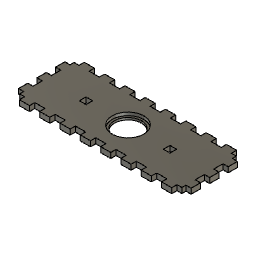
Top_of_Box-v3 (Autodesk Fusion 360 design; units mm, degrees)
Autodesk Fusion 360 part; units mm, degrees
sketch "Sketch1" plane through (0, 0, 0) normal (0, 0, 1) x (1, 0, 0)
  line L0 (0, 0) -> (165, 0)
  line L1 (165, 0) -> (165, 62)
  line L2 (165, 62) -> (0, 62)
  line L3 (0, 62) -> (0, 0)
  line L4 (0, 62) -> (9.7059, 62)
  line L5 (9.7059, 62) -> (9.7059, 57)
  line L6 (9.7059, 57) -> (0, 57)
  line L7 (0, 57) -> (0, 62)
  line L8 (9.7059, 62) -> (19.4118, 62)
  line L9 (19.4118, 62) -> (19.4118, 57)
  line L10 (19.4118, 57) -> (9.7059, 57)
  line L11 (9.7059, 57) -> (9.7059, 62)
  line L12 (19.4118, 62) -> (29.1176, 62)
  line L13 (29.1176, 62) -> (29.1176, 57)
  line L14 (29.1176, 57) -> (19.4118, 57)
  line L15 (19.4118, 57) -> (19.4118, 62)
  line L16 (29.1176, 62) -> (38.8235, 62)
  line L17 (38.8235, 62) -> (38.8235, 57)
  line L18 (38.8235, 57) -> (29.1176, 57)
  line L19 (29.1176, 57) -> (29.1176, 62)
  line L20 (38.8235, 62) -> (48.5294, 62)
  line L21 (48.5294, 62) -> (48.5294, 57)
  line L22 (48.5294, 57) -> (38.8235, 57)
  line L23 (38.8235, 57) -> (38.8235, 62)
  line L24 (48.5294, 62) -> (58.2353, 62)
  line L25 (58.2353, 62) -> (58.2353, 57)
  line L26 (58.2353, 57) -> (48.5294, 57)
  line L27 (48.5294, 57) -> (48.5294, 62)
  line L28 (58.2353, 62) -> (67.9412, 62)
  line L29 (67.9412, 62) -> (67.9412, 57)
  line L30 (67.9412, 57) -> (58.2353, 57)
  line L31 (58.2353, 57) -> (58.2353, 62)
  line L32 (67.9412, 62) -> (77.6471, 62)
  line L33 (77.6471, 62) -> (77.6471, 57)
  line L34 (77.6471, 57) -> (67.9412, 57)
  line L35 (67.9412, 57) -> (67.9412, 62)
  line L36 (77.6471, 62) -> (87.3529, 62)
  line L37 (87.3529, 62) -> (87.3529, 57)
  line L38 (87.3529, 57) -> (77.6471, 57)
  line L39 (77.6471, 57) -> (77.6471, 62)
  line L40 (87.3529, 62) -> (97.0588, 62)
  line L41 (97.0588, 62) -> (97.0588, 57)
  line L42 (97.0588, 57) -> (87.3529, 57)
  line L43 (87.3529, 57) -> (87.3529, 62)
  line L44 (97.0588, 62) -> (106.7647, 62)
  line L45 (106.7647, 62) -> (106.7647, 57)
  line L46 (106.7647, 57) -> (97.0588, 57)
  line L47 (97.0588, 57) -> (97.0588, 62)
  line L48 (106.7647, 62) -> (116.4706, 62)
  line L49 (116.4706, 62) -> (116.4706, 57)
  line L50 (116.4706, 57) -> (106.7647, 57)
  line L51 (106.7647, 57) -> (106.7647, 62)
  line L52 (116.4706, 62) -> (126.1765, 62)
  line L53 (126.1765, 62) -> (126.1765, 57)
  line L54 (126.1765, 57) -> (116.4706, 57)
  line L55 (116.4706, 57) -> (116.4706, 62)
  line L56 (126.1765, 62) -> (135.8824, 62)
  line L57 (135.8824, 62) -> (135.8824, 57)
  line L58 (135.8824, 57) -> (126.1765, 57)
  line L59 (126.1765, 57) -> (126.1765, 62)
  line L60 (135.8824, 62) -> (145.5882, 62)
  line L61 (145.5882, 62) -> (145.5882, 57)
  line L62 (145.5882, 57) -> (135.8824, 57)
  line L63 (135.8824, 57) -> (135.8824, 62)
  line L64 (145.5882, 62) -> (155.2941, 62)
  line L65 (155.2941, 62) -> (155.2941, 57)
  line L66 (155.2941, 57) -> (145.5882, 57)
  line L67 (145.5882, 57) -> (145.5882, 62)
  line L68 (155.2941, 62) -> (165, 62)
  line L69 (165, 62) -> (165, 57)
  line L70 (165, 57) -> (155.2941, 57)
  line L71 (155.2941, 57) -> (155.2941, 62)
  line L72 (0, 62) -> (5, 62)
  line L73 (5, 62) -> (5, 53.1429)
  line L74 (5, 53.1429) -> (0, 53.1429)
  line L75 (0, 53.1429) -> (0, 62)
  line L76 (5, 44.2857) -> (0, 44.2857)
  line L77 (5, 53.1429) -> (5, 44.2857)
  line L78 (0, 44.2857) -> (0, 53.1429)
  line L79 (0, 53.1429) -> (5, 53.1429)
  line L80 (5, 35.4286) -> (0, 35.4286)
  line L81 (5, 44.2857) -> (5, 35.4286)
  line L82 (0, 35.4286) -> (0, 44.2857)
  line L83 (0, 44.2857) -> (5, 44.2857)
  line L84 (5, 26.5714) -> (0, 26.5714)
  line L85 (5, 35.4286) -> (5, 26.5714)
  line L86 (0, 26.5714) -> (0, 35.4286)
  line L87 (0, 35.4286) -> (5, 35.4286)
  line L88 (5, 17.7143) -> (0, 17.7143)
  line L89 (5, 26.5714) -> (5, 17.7143)
  line L90 (0, 17.7143) -> (0, 26.5714)
  line L91 (0, 26.5714) -> (5, 26.5714)
  line L92 (5, 8.8571) -> (0, 8.8571)
  line L93 (5, 17.7143) -> (5, 8.8571)
  line L94 (0, 8.8571) -> (0, 17.7143)
  line L95 (0, 17.7143) -> (5, 17.7143)
  line L96 (5, 0) -> (0, 0)
  line L97 (5, 8.8571) -> (5, 0)
  line L98 (0, 0) -> (0, 8.8571)
  line L99 (0, 8.8571) -> (5, 8.8571)
  line L100 (0, 0) -> (9.7059, 0)
  line L101 (9.7059, 0) -> (9.7059, 5)
  line L102 (9.7059, 5) -> (0, 5)
  line L103 (0, 5) -> (0, 0)
  line L104 (9.7059, 0) -> (19.4118, 0)
  line L105 (19.4118, 0) -> (19.4118, 5)
  line L106 (9.7059, 5) -> (9.7059, 0)
  line L107 (19.4118, 5) -> (9.7059, 5)
  line L108 (19.4118, 0) -> (29.1176, 0)
  line L109 (29.1176, 0) -> (29.1176, 5)
  line L110 (19.4118, 5) -> (19.4118, 0)
  line L111 (29.1176, 5) -> (19.4118, 5)
  line L112 (29.1176, 0) -> (38.8235, 0)
  line L113 (38.8235, 0) -> (38.8235, 5)
  line L114 (29.1176, 5) -> (29.1176, 0)
  line L115 (38.8235, 5) -> (29.1176, 5)
  line L116 (38.8235, 0) -> (48.5294, 0)
  line L117 (48.5294, 0) -> (48.5294, 5)
  line L118 (38.8235, 5) -> (38.8235, 0)
  line L119 (48.5294, 5) -> (38.8235, 5)
  line L120 (48.5294, 0) -> (58.2353, 0)
  line L121 (58.2353, 0) -> (58.2353, 5)
  line L122 (48.5294, 5) -> (48.5294, 0)
  line L123 (58.2353, 5) -> (48.5294, 5)
  line L124 (58.2353, 0) -> (67.9412, 0)
  line L125 (67.9412, 0) -> (67.9412, 5)
  line L126 (58.2353, 5) -> (58.2353, 0)
  line L127 (67.9412, 5) -> (58.2353, 5)
  line L128 (67.9412, 0) -> (77.6471, 0)
  line L129 (77.6471, 0) -> (77.6471, 5)
  line L130 (67.9412, 5) -> (67.9412, 0)
  line L131 (77.6471, 5) -> (67.9412, 5)
  line L132 (77.6471, 0) -> (87.3529, 0)
  line L133 (87.3529, 0) -> (87.3529, 5)
  line L134 (77.6471, 5) -> (77.6471, 0)
  line L135 (87.3529, 5) -> (77.6471, 5)
  line L136 (87.3529, 0) -> (97.0588, 0)
  line L137 (97.0588, 0) -> (97.0588, 5)
  line L138 (87.3529, 5) -> (87.3529, 0)
  line L139 (97.0588, 5) -> (87.3529, 5)
  line L140 (97.0588, 0) -> (106.7647, 0)
  line L141 (106.7647, 0) -> (106.7647, 5)
  line L142 (97.0588, 5) -> (97.0588, 0)
  line L143 (106.7647, 5) -> (97.0588, 5)
  line L144 (106.7647, 0) -> (116.4706, 0)
  line L145 (116.4706, 0) -> (116.4706, 5)
  line L146 (106.7647, 5) -> (106.7647, 0)
  line L147 (116.4706, 5) -> (106.7647, 5)
  line L148 (116.4706, 0) -> (126.1765, 0)
  line L149 (126.1765, 0) -> (126.1765, 5)
  line L150 (116.4706, 5) -> (116.4706, 0)
  line L151 (126.1765, 5) -> (116.4706, 5)
  line L152 (126.1765, 0) -> (135.8824, 0)
  line L153 (135.8824, 0) -> (135.8824, 5)
  line L154 (126.1765, 5) -> (126.1765, 0)
  line L155 (135.8824, 5) -> (126.1765, 5)
  line L156 (135.8824, 0) -> (145.5882, 0)
  line L157 (145.5882, 0) -> (145.5882, 5)
  line L158 (135.8824, 5) -> (135.8824, 0)
  line L159 (145.5882, 5) -> (135.8824, 5)
  line L160 (145.5882, 0) -> (155.2941, 0)
  line L161 (155.2941, 0) -> (155.2941, 5)
  line L162 (145.5882, 5) -> (145.5882, 0)
  line L163 (155.2941, 5) -> (145.5882, 5)
  line L164 (155.2941, 0) -> (165, 0)
  line L165 (165, 0) -> (165, 5)
  line L166 (155.2941, 5) -> (155.2941, 0)
  line L167 (165, 5) -> (155.2941, 5)
  line L168 (165, 62) -> (160, 62)
  line L169 (160, 62) -> (160, 53.1429)
  line L170 (160, 53.1429) -> (165, 53.1429)
  line L171 (165, 53.1429) -> (165, 62)
  line L172 (160, 53.1429) -> (160, 44.2857)
  line L173 (160, 44.2857) -> (165, 44.2857)
  line L174 (160, 44.2857) -> (160, 35.4286)
  line L175 (160, 35.4286) -> (165, 35.4286)
  line L176 (160, 35.4286) -> (160, 26.5714)
  line L177 (160, 26.5714) -> (165, 26.5714)
  line L178 (160, 26.5714) -> (160, 17.7143)
  line L179 (160, 17.7143) -> (165, 17.7143)
  line L180 (160, 17.7143) -> (160, 8.8571)
  line L181 (160, 8.8571) -> (165, 8.8571)
  line L182 (160, 8.8571) -> (160, 0)
  line L183 (160, 0) -> (165, 0)
  dimension "d4" = 165
  dimension "d5" = 62
  dimension "d6" = 9.7059
  dimension "d7" = 5
  dimension "d10" = 155.2941
  dimension "d11" = 0
  dimension "d12" = 5
  dimension "d13" = 8.8571
  dimension "d16" = 0
  dimension "d17" = -53.1429
  dimension "d18" = 9.7059
  dimension "d19" = 5
  dimension "d22" = 155.2941
  dimension "d23" = 0
  dimension "d24" = 5
  dimension "d25" = 8.8571
  dimension "d28" = 0
  dimension "d29" = -53.1429
  constraint horizontal L0
  constraint vertical L1
  constraint horizontal L2
  constraint vertical L3
  constraint coincident L0.start L3.end
  constraint horizontal L4
  constraint vertical L5
  constraint horizontal L6
  constraint vertical L7
  constraint horizontal L72
  constraint vertical L73
  constraint horizontal L74
  constraint vertical L75
  measures "d4" distance of L0.start L0.end
  measures "d5" distance of L0.start L2.end
  measures "d6" distance of L2.end L4.end
  measures "d7" distance of L2.end L6.end
  measures "d12" distance of L2.end L72.end
  measures "d13" distance of L2.end L74.end
  measures "d18" distance of L0.start L100.end
  measures "d19" distance of L0.start L102.end
  measures "d24" distance of L1.end L168.end
  measures "d25" distance of L1.end L170.end
extrude "Extrude1" add sketch "Sketch1" along normal blind 5 contours L0 L101 L104 L105 L106 L107 L110 | L6 L10 L14 L18 L22 L26 L30 L34 L38 L42 L46 L50 L54 L58 L62 L66 L70 L73 L77 L81 L85 L89 L93 L97 L102 L107 L111 L115 L119 L123 L127 L131 L135 L139 L143 L147 L151 L155 L159 L163 L167 L169 L172 L174 L176 L178 L180 L182 | L3 L88 L92 L93 L94 L95 L99 | L0 L109 L112 L113 L114 L115 L118 | L3 L80 L84 L85 L86 L87 L91 | L0 L117 L120 L121 L122 L123 L126 | L3 L74 L76 L77 L78 L79 L83 | L0 L125 L128 L129 L130 L131 L134 | L0 L133 L136 L137 L138 L139 L142 | L2 L5 L8 L9 L10 L11 L15 | L0 L141 L144 L145 L146 L147 L150 | L2 L13 L16 L17 L18 L19 L23 | L0 L149 L152 L153 L154 L155 L158 | L2 L21 L24 L25 L26 L27 L31 | L0 L157 L160 L161 L162 L163 L166 | L2 L29 L32 L33 L34 L35 L39 | L2 L37 L40 L41 L42 L43 L47 | L1 L179 L180 L181 | L2 L45 L48 L49 L50 L51 L55 | L1 L175 L176 L177 | L2 L53 L56 L57 L58 L59 L63 | L1 L170 L172 L173 | L2 L61 L64 L65 L66 L67 L71
sketch "Sketch2" plane through (0, 0, 5) normal (0, 0, 1) x (-1, 0, 0)
  line L0 (-165, -8.8571) -> (-165, -17.7143)
  line L1 (-165, -17.7143) -> (-160, -17.7143)
  line L2 (-160, -17.7143) -> (-160, -26.5714)
  line L3 (-160, -26.5714) -> (-165, -26.5714)
  line L4 (-165, -26.5714) -> (-165, -35.4286)
  line L5 (-165, -35.4286) -> (-160, -35.4286)
  line L6 (-160, -35.4286) -> (-160, -44.2857)
  line L7 (-160, -44.2857) -> (-165, -44.2857)
  line L8 (-165, -44.2857) -> (-165, -53.1429)
  line L9 (-165, -53.1429) -> (-160, -53.1429)
  line L10 (-160, -53.1429) -> (-160, -57)
  line L11 (-160, -57) -> (-155.2941, -57)
  line L12 (-155.2941, -57) -> (-155.2941, -62)
  line L13 (-155.2941, -62) -> (-145.5882, -62)
  line L14 (-145.5882, -62) -> (-145.5882, -57)
  line L15 (-145.5882, -57) -> (-135.8824, -57)
  line L16 (-135.8824, -57) -> (-135.8824, -62)
  line L17 (-135.8824, -62) -> (-126.1765, -62)
  line L18 (-126.1765, -62) -> (-126.1765, -57)
  line L19 (-126.1765, -57) -> (-116.4706, -57)
  line L20 (-116.4706, -57) -> (-116.4706, -62)
  line L21 (-116.4706, -62) -> (-106.7647, -62)
  line L22 (-106.7647, -62) -> (-106.7647, -57)
  line L23 (-106.7647, -57) -> (-97.0588, -57)
  line L24 (-97.0588, -57) -> (-97.0588, -62)
  line L25 (-97.0588, -62) -> (-87.3529, -62)
  line L26 (-87.3529, -62) -> (-87.3529, -57)
  line L27 (-87.3529, -57) -> (-77.6471, -57)
  line L28 (-77.6471, -57) -> (-77.6471, -62)
  line L29 (-77.6471, -62) -> (-67.9412, -62)
  line L30 (-67.9412, -62) -> (-67.9412, -57)
  line L31 (-67.9412, -57) -> (-58.2353, -57)
  line L32 (-58.2353, -57) -> (-58.2353, -62)
  line L33 (-58.2353, -62) -> (-48.5294, -62)
  line L34 (-48.5294, -62) -> (-48.5294, -57)
  line L35 (-48.5294, -57) -> (-38.8235, -57)
  line L36 (-38.8235, -57) -> (-38.8235, -62)
  line L37 (-38.8235, -62) -> (-29.1176, -62)
  line L38 (-29.1176, -62) -> (-29.1176, -57)
  line L39 (-29.1176, -57) -> (-19.4118, -57)
  line L40 (-19.4118, -57) -> (-19.4118, -62)
  line L41 (-19.4118, -62) -> (-9.7059, -62)
  line L42 (-9.7059, -62) -> (-9.7059, -57)
  line L43 (-9.7059, -57) -> (-5, -57)
  line L44 (-5, -57) -> (-5, -53.1429)
  line L45 (-5, -53.1429) -> (0, -53.1429)
  line L46 (0, -53.1429) -> (0, -44.2857)
  line L47 (0, -44.2857) -> (-5, -44.2857)
  line L48 (-5, -44.2857) -> (-5, -35.4286)
  line L49 (-5, -35.4286) -> (0, -35.4286)
  line L50 (0, -35.4286) -> (0, -26.5714)
  line L51 (0, -26.5714) -> (-5, -26.5714)
  line L52 (-5, -26.5714) -> (-5, -17.7143)
  line L53 (-5, -17.7143) -> (0, -17.7143)
  line L54 (0, -17.7143) -> (0, -8.8571)
  line L55 (0, -8.8571) -> (-5, -8.8571)
  line L56 (-5, -8.8571) -> (-5, -5)
  line L57 (-5, -5) -> (-9.7059, -5)
  line L58 (-9.7059, -5) -> (-9.7059, 0)
  line L59 (-9.7059, 0) -> (-19.4118, 0)
  line L60 (-19.4118, 0) -> (-19.4118, -5)
  line L61 (-19.4118, -5) -> (-29.1176, -5)
  line L62 (-29.1176, -5) -> (-29.1176, 0)
  line L63 (-29.1176, 0) -> (-38.8235, 0)
  line L64 (-38.8235, 0) -> (-38.8235, -5)
  line L65 (-38.8235, -5) -> (-48.5294, -5)
  line L66 (-48.5294, -5) -> (-48.5294, 0)
  line L67 (-48.5294, 0) -> (-58.2353, 0)
  line L68 (-58.2353, 0) -> (-58.2353, -5)
  line L69 (-58.2353, -5) -> (-67.9412, -5)
  line L70 (-67.9412, -5) -> (-67.9412, 0)
  line L71 (-67.9412, 0) -> (-77.6471, 0)
  line L72 (-77.6471, 0) -> (-77.6471, -5)
  line L73 (-77.6471, -5) -> (-87.3529, -5)
  line L74 (-87.3529, -5) -> (-87.3529, 0)
  line L75 (-87.3529, 0) -> (-97.0588, 0)
  line L76 (-97.0588, 0) -> (-97.0588, -5)
  line L77 (-97.0588, -5) -> (-106.7647, -5)
  line L78 (-106.7647, -5) -> (-106.7647, 0)
  line L79 (-106.7647, 0) -> (-116.4706, 0)
  line L80 (-116.4706, 0) -> (-116.4706, -5)
  line L81 (-116.4706, -5) -> (-126.1765, -5)
  line L82 (-126.1765, -5) -> (-126.1765, 0)
  line L83 (-126.1765, 0) -> (-135.8824, 0)
  line L84 (-135.8824, 0) -> (-135.8824, -5)
  line L85 (-135.8824, -5) -> (-145.5882, -5)
  line L86 (-145.5882, -5) -> (-145.5882, 0)
  line L87 (-145.5882, 0) -> (-155.2941, 0)
  line L88 (-155.2941, 0) -> (-155.2941, -5)
  line L89 (-155.2941, -5) -> (-160, -5)
  line L90 (-160, -5) -> (-160, -8.8571)
  line L91 (-160, -8.8571) -> (-165, -8.8571)
  line L92 (0, -31) -> (-82.5, -31) construction
  circle A0 centre (-82.5, -31) radius 13
  dimension "d36" = 82.5
  dimension "d38" = 26
  constraint midpoint L50 L92.start
  constraint perpendicular L50 L92
  constraint coincident L92.end A0.centre
  measures "d36" distance of L92.start L92.end
  measures "d38" diameter of A0
extrude "Extrude2" cut sketch "Sketch2" against normal up to surface (5 mm away) contours A0
sketch "Sketch3" plane through (0, 0, 5) normal (0, 0, 1) x (-1, 0, 0)
  circle A0 centre (-82.5, -31) radius 13
  line L0 (-165, -8.8571) -> (-165, -17.7143)
  line L1 (-165, -17.7143) -> (-160, -17.7143)
  line L2 (-160, -17.7143) -> (-160, -26.5714)
  line L3 (-160, -26.5714) -> (-165, -26.5714)
  line L4 (-165, -26.5714) -> (-165, -35.4286)
  line L5 (-165, -35.4286) -> (-160, -35.4286)
  line L6 (-160, -35.4286) -> (-160, -44.2857)
  line L7 (-160, -44.2857) -> (-165, -44.2857)
  line L8 (-165, -44.2857) -> (-165, -53.1429)
  line L9 (-165, -53.1429) -> (-160, -53.1429)
  line L10 (-160, -53.1429) -> (-160, -57)
  line L11 (-160, -57) -> (-155.2941, -57)
  line L12 (-155.2941, -57) -> (-155.2941, -62)
  line L13 (-155.2941, -62) -> (-145.5882, -62)
  line L14 (-145.5882, -62) -> (-145.5882, -57)
  line L15 (-145.5882, -57) -> (-135.8824, -57)
  line L16 (-135.8824, -57) -> (-135.8824, -62)
  line L17 (-135.8824, -62) -> (-126.1765, -62)
  line L18 (-126.1765, -62) -> (-126.1765, -57)
  line L19 (-126.1765, -57) -> (-116.4706, -57)
  line L20 (-116.4706, -57) -> (-116.4706, -62)
  line L21 (-116.4706, -62) -> (-106.7647, -62)
  line L22 (-106.7647, -62) -> (-106.7647, -57)
  line L23 (-106.7647, -57) -> (-97.0588, -57)
  line L24 (-97.0588, -57) -> (-97.0588, -62)
  line L25 (-97.0588, -62) -> (-87.3529, -62)
  line L26 (-87.3529, -62) -> (-87.3529, -57)
  line L27 (-87.3529, -57) -> (-77.6471, -57)
  line L28 (-77.6471, -57) -> (-77.6471, -62)
  line L29 (-77.6471, -62) -> (-67.9412, -62)
  line L30 (-67.9412, -62) -> (-67.9412, -57)
  line L31 (-67.9412, -57) -> (-58.2353, -57)
  line L32 (-58.2353, -57) -> (-58.2353, -62)
  line L33 (-58.2353, -62) -> (-48.5294, -62)
  line L34 (-48.5294, -62) -> (-48.5294, -57)
  line L35 (-48.5294, -57) -> (-38.8235, -57)
  line L36 (-38.8235, -57) -> (-38.8235, -62)
  line L37 (-38.8235, -62) -> (-29.1176, -62)
  line L38 (-29.1176, -62) -> (-29.1176, -57)
  line L39 (-29.1176, -57) -> (-19.4118, -57)
  line L40 (-19.4118, -57) -> (-19.4118, -62)
  line L41 (-19.4118, -62) -> (-9.7059, -62)
  line L42 (-9.7059, -62) -> (-9.7059, -57)
  line L43 (-9.7059, -57) -> (-5, -57)
  line L44 (-5, -57) -> (-5, -53.1429)
  line L45 (-5, -53.1429) -> (0, -53.1429)
  line L46 (0, -53.1429) -> (0, -44.2857)
  line L47 (0, -44.2857) -> (-5, -44.2857)
  line L48 (-5, -44.2857) -> (-5, -35.4286)
  line L49 (-5, -35.4286) -> (0, -35.4286)
  line L50 (0, -35.4286) -> (0, -26.5714)
  line L51 (0, -26.5714) -> (-5, -26.5714)
  line L52 (-5, -26.5714) -> (-5, -17.7143)
  line L53 (-5, -17.7143) -> (0, -17.7143)
  line L54 (0, -17.7143) -> (0, -8.8571)
  line L55 (0, -8.8571) -> (-5, -8.8571)
  line L56 (-5, -8.8571) -> (-5, -5)
  line L57 (-5, -5) -> (-9.7059, -5)
  line L58 (-9.7059, -5) -> (-9.7059, 0)
  line L59 (-9.7059, 0) -> (-19.4118, 0)
  line L60 (-19.4118, 0) -> (-19.4118, -5)
  line L61 (-19.4118, -5) -> (-29.1176, -5)
  line L62 (-29.1176, -5) -> (-29.1176, 0)
  line L63 (-29.1176, 0) -> (-38.8235, 0)
  line L64 (-38.8235, 0) -> (-38.8235, -5)
  line L65 (-38.8235, -5) -> (-48.5294, -5)
  line L66 (-48.5294, -5) -> (-48.5294, 0)
  line L67 (-48.5294, 0) -> (-58.2353, 0)
  line L68 (-58.2353, 0) -> (-58.2353, -5)
  line L69 (-58.2353, -5) -> (-67.9412, -5)
  line L70 (-67.9412, -5) -> (-67.9412, 0)
  line L71 (-67.9412, 0) -> (-77.6471, 0)
  line L72 (-77.6471, 0) -> (-77.6471, -5)
  line L73 (-77.6471, -5) -> (-87.3529, -5)
  line L74 (-87.3529, -5) -> (-87.3529, 0)
  line L75 (-87.3529, 0) -> (-97.0588, 0)
  line L76 (-97.0588, 0) -> (-97.0588, -5)
  line L77 (-97.0588, -5) -> (-106.7647, -5)
  line L78 (-106.7647, -5) -> (-106.7647, 0)
  line L79 (-106.7647, 0) -> (-116.4706, 0)
  line L80 (-116.4706, 0) -> (-116.4706, -5)
  line L81 (-116.4706, -5) -> (-126.1765, -5)
  line L82 (-126.1765, -5) -> (-126.1765, 0)
  line L83 (-126.1765, 0) -> (-135.8824, 0)
  line L84 (-135.8824, 0) -> (-135.8824, -5)
  line L85 (-135.8824, -5) -> (-145.5882, -5)
  line L86 (-145.5882, -5) -> (-145.5882, 0)
  line L87 (-145.5882, 0) -> (-155.2941, 0)
  line L88 (-155.2941, 0) -> (-155.2941, -5)
  line L89 (-155.2941, -5) -> (-160, -5)
  line L90 (-160, -5) -> (-160, -8.8571)
  line L91 (-160, -8.8571) -> (-165, -8.8571)
  line L92 (0, -31) -> (-82.5, -31) construction
  circle A1 centre (-82.5, -31) radius 15.125
  dimension "d41" = 82.5
  dimension "d42" = 30.25
  constraint midpoint L50 L92.start
  constraint perpendicular L50 L92
  constraint coincident A0.centre L92.end
  measures "d41" distance of L92.start A0.centre
  measures "d42" diameter of A1
extrude "Extrude3" cut sketch "Sketch3" against normal blind 3 contours A1
sketch "Sketch4" plane through (0, 0, 5) normal (0, 0, 1) x (-1, 0, 0)
  circle A0 centre (-82.5, -31) radius 15.125
  line L0 (-165, -8.8571) -> (-165, -17.7143)
  line L1 (-165, -17.7143) -> (-160, -17.7143)
  line L2 (-160, -17.7143) -> (-160, -26.5714)
  line L3 (-160, -26.5714) -> (-165, -26.5714)
  line L4 (-165, -26.5714) -> (-165, -35.4286)
  line L5 (-165, -35.4286) -> (-160, -35.4286)
  line L6 (-160, -35.4286) -> (-160, -44.2857)
  line L7 (-160, -44.2857) -> (-165, -44.2857)
  line L8 (-165, -44.2857) -> (-165, -53.1429)
  line L9 (-165, -53.1429) -> (-160, -53.1429)
  line L10 (-160, -53.1429) -> (-160, -57)
  line L11 (-160, -57) -> (-155.2941, -57)
  line L12 (-155.2941, -57) -> (-155.2941, -62)
  line L13 (-155.2941, -62) -> (-145.5882, -62)
  line L14 (-145.5882, -62) -> (-145.5882, -57)
  line L15 (-145.5882, -57) -> (-135.8824, -57)
  line L16 (-135.8824, -57) -> (-135.8824, -62)
  line L17 (-135.8824, -62) -> (-126.1765, -62)
  line L18 (-126.1765, -62) -> (-126.1765, -57)
  line L19 (-126.1765, -57) -> (-116.4706, -57)
  line L20 (-116.4706, -57) -> (-116.4706, -62)
  line L21 (-116.4706, -62) -> (-106.7647, -62)
  line L22 (-106.7647, -62) -> (-106.7647, -57)
  line L23 (-106.7647, -57) -> (-97.0588, -57)
  line L24 (-97.0588, -57) -> (-97.0588, -62)
  line L25 (-97.0588, -62) -> (-87.3529, -62)
  line L26 (-87.3529, -62) -> (-87.3529, -57)
  line L27 (-87.3529, -57) -> (-77.6471, -57)
  line L28 (-77.6471, -57) -> (-77.6471, -62)
  line L29 (-77.6471, -62) -> (-67.9412, -62)
  line L30 (-67.9412, -62) -> (-67.9412, -57)
  line L31 (-67.9412, -57) -> (-58.2353, -57)
  line L32 (-58.2353, -57) -> (-58.2353, -62)
  line L33 (-58.2353, -62) -> (-48.5294, -62)
  line L34 (-48.5294, -62) -> (-48.5294, -57)
  line L35 (-48.5294, -57) -> (-38.8235, -57)
  line L36 (-38.8235, -57) -> (-38.8235, -62)
  line L37 (-38.8235, -62) -> (-29.1176, -62)
  line L38 (-29.1176, -62) -> (-29.1176, -57)
  line L39 (-29.1176, -57) -> (-19.4118, -57)
  line L40 (-19.4118, -57) -> (-19.4118, -62)
  line L41 (-19.4118, -62) -> (-9.7059, -62)
  line L42 (-9.7059, -62) -> (-9.7059, -57)
  line L43 (-9.7059, -57) -> (-5, -57)
  line L44 (-5, -57) -> (-5, -53.1429)
  line L45 (-5, -53.1429) -> (0, -53.1429)
  line L46 (0, -53.1429) -> (0, -44.2857)
  line L47 (0, -44.2857) -> (-5, -44.2857)
  line L48 (-5, -44.2857) -> (-5, -35.4286)
  line L49 (-5, -35.4286) -> (0, -35.4286)
  line L50 (0, -35.4286) -> (0, -26.5714)
  line L51 (0, -26.5714) -> (-5, -26.5714)
  line L52 (-5, -26.5714) -> (-5, -17.7143)
  line L53 (-5, -17.7143) -> (0, -17.7143)
  line L54 (0, -17.7143) -> (0, -8.8571)
  line L55 (0, -8.8571) -> (-5, -8.8571)
  line L56 (-5, -8.8571) -> (-5, -5)
  line L57 (-5, -5) -> (-9.7059, -5)
  line L58 (-9.7059, -5) -> (-9.7059, 0)
  line L59 (-9.7059, 0) -> (-19.4118, 0)
  line L60 (-19.4118, 0) -> (-19.4118, -5)
  line L61 (-19.4118, -5) -> (-29.1176, -5)
  line L62 (-29.1176, -5) -> (-29.1176, 0)
  line L63 (-29.1176, 0) -> (-38.8235, 0)
  line L64 (-38.8235, 0) -> (-38.8235, -5)
  line L65 (-38.8235, -5) -> (-48.5294, -5)
  line L66 (-48.5294, -5) -> (-48.5294, 0)
  line L67 (-48.5294, 0) -> (-58.2353, 0)
  line L68 (-58.2353, 0) -> (-58.2353, -5)
  line L69 (-58.2353, -5) -> (-67.9412, -5)
  line L70 (-67.9412, -5) -> (-67.9412, 0)
  line L71 (-67.9412, 0) -> (-77.6471, 0)
  line L72 (-77.6471, 0) -> (-77.6471, -5)
  line L73 (-77.6471, -5) -> (-87.3529, -5)
  line L74 (-87.3529, -5) -> (-87.3529, 0)
  line L75 (-87.3529, 0) -> (-97.0588, 0)
  line L76 (-97.0588, 0) -> (-97.0588, -5)
  line L77 (-97.0588, -5) -> (-106.7647, -5)
  line L78 (-106.7647, -5) -> (-106.7647, 0)
  line L79 (-106.7647, 0) -> (-116.4706, 0)
  line L80 (-116.4706, 0) -> (-116.4706, -5)
  line L81 (-116.4706, -5) -> (-126.1765, -5)
  line L82 (-126.1765, -5) -> (-126.1765, 0)
  line L83 (-126.1765, 0) -> (-135.8824, 0)
  line L84 (-135.8824, 0) -> (-135.8824, -5)
  line L85 (-135.8824, -5) -> (-145.5882, -5)
  line L86 (-145.5882, -5) -> (-145.5882, 0)
  line L87 (-145.5882, 0) -> (-155.2941, 0)
  line L88 (-155.2941, 0) -> (-155.2941, -5)
  line L89 (-155.2941, -5) -> (-160, -5)
  line L90 (-160, -5) -> (-160, -8.8571)
  line L91 (-160, -8.8571) -> (-165, -8.8571)
  line L92 (-165, -31) -> (-97.625, -31) construction
  line L93 (-97.625, -31) -> (-122.625, -31) construction
  line L94 (-125.775, -34.15) -> (-119.475, -34.15)
  line L95 (-119.475, -34.15) -> (-119.475, -27.85)
  line L96 (-119.475, -27.85) -> (-125.775, -27.85)
  line L97 (-125.775, -27.85) -> (-125.775, -34.15)
  line L98 (-125.775, -34.15) -> (-119.475, -27.85) construction
  line L99 (-119.475, -34.15) -> (-125.775, -27.85) construction
  line L100 (0, -31) -> (-67.375, -31) construction
  line L101 (-67.375, -31) -> (-42.375, -31) construction
  line L102 (-39.225, -27.85) -> (-45.525, -27.85)
  line L103 (-45.525, -27.85) -> (-45.525, -34.15)
  line L104 (-45.525, -34.15) -> (-39.225, -34.15)
  line L105 (-39.225, -34.15) -> (-39.225, -27.85)
  line L106 (-39.225, -27.85) -> (-45.525, -34.15) construction
  line L107 (-45.525, -27.85) -> (-39.225, -34.15) construction
  point P0 (-122.625, -31)
  point P1 (-42.375, -31)
  dimension "d48" = 25
  dimension "d49" = 6.3
  dimension "d50" = 6.3
  dimension "d51" = 25
  dimension "d52" = 6.3
  dimension "d53" = 6.3
  constraint midpoint L4 L92.start
  constraint coincident A0 L92.end
  constraint perpendicular L4 L92
  constraint parallel L92 L93
  constraint horizontal L94
  constraint perpendicular L94 L95
  constraint parallel L94 L96
  constraint parallel L95 L97
  constraint coincident L98 P0
  constraint coincident L99 P0
  constraint coincident P0 L93.end
  constraint midpoint L50 L100.start
  constraint coincident A0 L100.end
  constraint perpendicular L50 L100
  constraint perpendicular L50 L101
  constraint horizontal L102
  constraint perpendicular L102 L103
  constraint parallel L102 L104
  constraint parallel L103 L105
  constraint coincident L106 P1
  constraint coincident L107 P1
  constraint coincident P1 L101.end
  measures "d48" distance of L92.end P0
  measures "d49" distance of L95.end L96.end
  measures "d50" distance of L94.end L95.end
  measures "d51" distance of L100.end P1
  measures "d52" distance of L103.end L104.end
  measures "d53" distance of L102.end L103.end
extrude "Extrude4" cut sketch "Sketch4" against normal up to surface (5 mm away) contours L94 L95 L96 L97 | L102 L103 L104 L105
equation "box_length = 165 mm"
equation "box_width = 62 mm"
equation "box_depth = 5 mm"
equation "d4 = box_length"
equation "d5 = box_width"
equation "d6 = box_length / 17"
equation "d7 = box_depth"
equation "d10 = box_length - box_length / 17"
equation "d12 = box_depth"
equation "d13 = box_width / 7"
equation "d17 = -box_width + box_width / 7"
equation "d18 = box_length / 17"
equation "d19 = box_depth"
equation "d22 = box_length - box_length / 17"
equation "d24 = box_depth"
equation "d25 = box_width / 7"
equation "d29 = -box_width + box_width / 7"
equation "d30 = box_depth"
equation "buzzer_diam = 30.25 mm"
equation "d36 = box_length / 2"
equation "buzzer_hole_diam = 26 mm"
equation "d38 = buzzer_hole_diam"
equation "d41 = box_length / 2"
equation "d42 = buzzer_diam"
equation "d43 = -box_depth + 2 mm"
equation "button_depth = 3.5 mm"
equation "button_width = 6.3 mm"
equation "button_hole_width = 4.5 mm"
equation "d49 = button_width"
equation "d50 = button_width"
equation "d52 = button_width"
equation "d53 = button_width"
